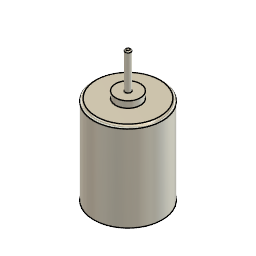
Motor (Autodesk Fusion 360 design; units mm, degrees)
part number: 2026-04-29-15-15-11-986
Autodesk Fusion 360 part; units mm, degrees
sketch "Sketch1" plane through (0, 0, 0) normal (0, 1, 0) x (1, 0, 0)
  circle A0 centre (0, 0) radius 13.85
  dimension "d1" = 27.7
  constraint coincident A0.centre origin
  measures "d1" diameter of A0
extrude "Extrude1" add sketch "Sketch1" along normal blind 38
sketch "Sketch2" plane through (0, 38, 0) normal (0, 1, 0) x (-1, 0, 0)
  circle A0 centre (0, 0) radius 13.85
  circle A1 centre (0, 0) radius 5
  dimension "d4" = 10
  constraint coincident A0.centre A1.centre
  measures "d4" diameter of A1
extrude "Extrude2" add sketch "Sketch2" along normal blind 2.6 contours A1
sketch "Sketch3" plane through (0, 40.6, 0) normal (0, 1, 0) x (-1, 0, 0)
  circle A0 centre (0, 0) radius 5
  circle A1 centre (0, 0) radius 1.15
  dimension "d7" = 2.3
  constraint coincident A0.centre A1.centre
  measures "d7" diameter of A1
extrude "Extrude3" add sketch "Sketch3" along normal blind 14.55 contours A1
sketch "Sketch4" plane through (0, 0, 0) normal (0, -1, 0) x (1, 0, 0)
  circle A0 centre (0, 0) radius 13.85
  circle A1 centre (0, 0) radius 5
  dimension "d10" = 10
  constraint coincident A0.centre A1.centre
  measures "d10" diameter of A1
extrude "Extrude4" cut sketch "Sketch4" against normal blind 2.2
fillet "Fillet1" radius 1 1 edges at (-12.9127, 38, 5.0084)
fillet "Fillet2" radius 0.5 1 edges at (1.0722, 55.15, -0.4159)
fillet "Fillet3" radius 0.1 2 edges at (-12.9127, 2.2, 5.0084) (-4.6616, 0, -1.8081)
